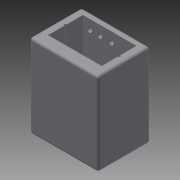
# Autodesk Inventor part: Part1
Saved by Autodesk Inventor 2014 SP1 (Build 180222100, 222)
## iProperties
Created: 2013-12-01
Part Number: Part1
Material: Generic
Document SubType Name: Modeling
Designer: Tim
Density: 1 g/cm^3
Appearance: Default
Author: Tim
Autodesk Inventor part; units mm, degrees
ref_plane "YZ Plane" through (0, 0, 0) normal (1, 0, 0) x (0, 1, 0)
ref_plane "XZ Plane" through (0, 0, 0) normal (0, 1, 0) x (-1, 0, 0)
ref_plane "XY Plane" through (0, 0, 0) normal (0, 0, 1) x (1, 0, 0)
sketch "Sketch1" plane through (0, 0, 0) normal (0, 1, 0) x (-1, 0, 0)
  line L0 (27.4909, -23.2831) -> (-26.5091, -23.2831)
  line L1 (-26.5091, -23.2831) -> (-26.5091, 42.2169)
  line L2 (-26.5091, 42.2169) -> (27.4909, 42.2169)
  line L3 (27.4909, 42.2169) -> (27.4909, -23.2831)
  point P0 (0, 0)
  dimension "d0" = 54
  dimension "d1" = 65.5
  constraints: 8 end point, 2 parallel, 1 horizontal, 1 perpendicular
  measures "d0" distance between parallel lines of L3 L1
  measures "d1" distance between parallel lines of L0 L2
extrude "Extrusion1" add sketch "Sketch1" along normal blind 41
sketch "Sketch2" plane through (-27.4909, 0, 42.2169) normal (0, 0, 1) x (1, 0, 0)
  line L0 (54, 0) -> (0, 0) projected
  line L1 (54, 0) -> (54, 41) projected
  line L2 (0, 41) -> (54, 41) projected
  line L3 (0, 0) -> (0, 41) projected
  line L4 (6, 36) -> (48, 36)
  line L5 (48, 36) -> (48, 5)
  line L6 (48, 5) -> (6, 5)
  line L7 (6, 5) -> (6, 36)
  line L8 (5, 23) -> (49, 23)
  line L9 (49, 23) -> (49, 21.5)
  line L10 (49, 21.5) -> (5, 21.5)
  line L11 (5, 21.5) -> (5, 23)
  point P0 (27.4909, 0)
  dimension "d4" = 42
  dimension "d5" = 31
  dimension "d6" = 5
  dimension "d7" = 6
  dimension "d8" = 6
  dimension "d9" = 1
  dimension "d10" = 1
  dimension "d11" = 13
  dimension "d12" = 1.5
  dimension "d13" = 5
  constraints: 16 end point, 4 parallel, 2 horizontal, 2 perpendicular
  measures "d4" distance between parallel lines of L5 L7
  measures "d5" distance between parallel lines of L6 L4
  measures "d6" distance between parallel lines of L4 L2
  measures "d7" distance between parallel lines of L1 L5
  measures "d8" distance between parallel lines of L3 L7
  measures "d9" distance between parallel lines of L7 L11
  measures "d10" distance between parallel lines of L9 L5
  measures "d11" distance between parallel lines of L4 L8
  measures "d12" distance between parallel lines of L8 L10
  measures "d13" distance between parallel lines of L0 L6
extrude "Extrusion2" cut sketch "Sketch2" against normal blind 60.5 contours L4 L5 L8 L7 | L8 L5 L10 L7 | L7 L10 L11 L8 | L8 L9 L10 L5 | L10 L5 L6 L7
sketch "Sketch3" plane through (0, 41, 0) normal (0, 1, 0) x (1, 0, 0)
  line L0 (26.5091, 23.2831) -> (-27.4909, 23.2831) projected
  line L1 (26.5091, -42.2169) -> (26.5091, 23.2831) projected
  line L2 (-6.9909, -5.7169) -> (18.5091, -5.7169)
  line L3 (18.5091, -5.7169) -> (18.5091, 15.2831)
  line L4 (18.5091, 15.2831) -> (-6.9909, 15.2831)
  line L5 (-6.9909, 15.2831) -> (-6.9909, -5.7169)
  point P0 (0, 0)
  dimension "d16" = 33.5
  dimension "d17" = 29
  dimension "d18" = 8
  dimension "d19" = 8
  constraints: 8 end point, 2 parallel, 1 horizontal, 1 perpendicular
  measures "d16" distance between parallel lines of L1 L5
  measures "d17" distance between parallel lines of L0 L2
  measures "d18" distance between parallel lines of L0 L4
  measures "d19" distance between parallel lines of L1 L3
extrude "Extrusion3" cut sketch "Sketch3" against normal blind 5
sketch "Sketch4" plane through (-21.4909, 5, 42.2169) normal (0, 1, 0) x (1, 0, 0)
  line L0 (0, 0) -> (0, 60.5) projected
  line L1 (0, 8) -> (42, 8)
  line L2 (42, 8) -> (42, 0)
  line L3 (42, 0) -> (0, 0)
  line L4 (0, 0) -> (0, 8)
  point P0 (21.4909, 42.2169)
  dimension "d22" = 8
  constraints: 8 end point, 2 parallel, 1 horizontal, 1 perpendicular, 1 point on line
  measures "d22" distance between parallel lines of L3 L1
extrude "Extrusion4" add sketch "Sketch4" along normal blind 5 separate body
sketch "Sketch5" plane through (0, 41, 0) normal (0, 1, 0) x (1, 0, 0)
  line L0 (26.5091, 23.2831) -> (-27.4909, 23.2831) projected
  line L1 (-27.4909, 23.2831) -> (-27.4909, -42.2169) projected
  circle A0 centre (-16.4909, -34.7169) radius 2
  circle A1 centre (-8.4909, -34.7169) radius 2
  circle A2 centre (0.5091, -34.7169) radius 2
  point P0 (0, 0)
  dimension "d25" = 11
  dimension "d26" = 19
  dimension "d27" = 28
  dimension "d30" = 58
  dimension "d31" = 58
  dimension "d32" = 58
  dimension "d33" = 4
  dimension "d34" = 4
  dimension "d35" = 4
  constraints: 3 centre point
  measures "d25" distance from line of L1 A0.centre
  measures "d26" distance from line of A1.centre L1
  measures "d27" distance from line of A2.centre L1
  measures "d30" distance from line of L0 A0.centre
  measures "d31" distance from line of L0 A1.centre
  measures "d32" distance from line of L0 A2.centre
  measures "d33" diameter of A1
  measures "d34" diameter of A2
  measures "d35" diameter of A0
extrude "Extrusion5" cut sketch "Sketch5" against normal blind 5 bodies 1
fillet "Fillet1" radius 5 1 edges at (-6.9909, 38.5, 5.7169)
fillet "Fillet2" radius 5 1 edges at (18.5091, 38.5, 5.7169)
fillet "Fillet3" radius 2 1 edges at (26.5091, 20.5, -23.2831)
fillet "Fillet4" radius 2 1 edges at (-27.4909, 20.5, -23.2831)
fillet "Fillet5" radius 2 5 edges at (-0.4909, 41, -23.2831) (-26.9051, 41, -22.6973) (-27.4909, 41, 10.4669) (25.9233, 41, -22.6973) (26.5091, 41, 10.4669)
fillet "Fillet6" radius 2 5 edges at (-0.4909, 0, -23.2831) (25.9233, 0, -22.6973) (26.5091, 0, 10.4669) (-26.9051, 0, -22.6973) (-27.4909, 0, 10.4669)
fillet "Fillet7" radius 2 8 edges at (-27.4909, 20.5, 42.2169) (-26.9051, 40.4142, 42.2169) (-0.4909, 41, 42.2169) (25.9233, 40.4142, 42.2169) (26.5091, 20.5, 42.2169) (25.9233, 0.5858, 42.2169) (-0.4909, 0, 42.2169) (-26.9051, 0.5858, 42.2169)
fillet "Fillet8" radius 2 5 edges at (5.7591, 41, 5.7169) (-5.5264, 41, 4.2524) (-6.9909, 41, -7.2831) (17.0446, 41, 4.2524) (18.5091, 41, -7.2831)
fillet "Fillet9" radius 1 3 edges at (-10.4909, 41, 34.7169) (-1.4909, 41, 34.7169) (-18.4909, 41, 34.7169)
fillet "Fillet10" radius 1 3 edges at (-7.9909, 41, -15.2831) (5.7591, 41, -15.2831) (19.5091, 41, -15.2831)
fillet "Fillet11" radius 2 1 edges at (-0.4909, 10, 42.2169)
sketch "Sketch6" plane through (24.5091, 39, -23.2831) normal (0, 0, -1) x (-1, 0, 0)
  line L0 (50, 0) -> (50, -37) projected
  line L1 (0, 0) -> (50, 0) projected
  line L2 (0, -37) -> (0, 0) projected
  line L3 (6, -15) -> (44, -15) construction
  line L4 (44, -15) -> (44, -20) construction
  line L5 (44, -20) -> (6, -20) construction
  line L6 (6, -20) -> (6, -15) construction
  line L7 (7.1714, -18.5227) -> (7.1714, -15.4368)
  line L8 (7.1714, -15.4368) -> (5.9972, -15.4368)
  line L9 (5.9972, -15.4368) -> (5.9972, -15.0227)
  line L10 (5.9972, -15.0227) -> (8.8108, -15.0227)
  line L11 (8.8108, -15.0227) -> (8.8108, -15.4368)
  line L12 (8.8108, -15.4368) -> (7.6365, -15.4368)
  line L13 (7.6365, -15.4368) -> (7.6365, -18.5227)
  line L14 (7.6365, -18.5227) -> (7.1714, -18.5227)
  line L15 (9.5823, -18.5227) -> (9.1398, -18.5227)
  line L16 (9.1398, -18.5227) -> (9.1398, -15.8963)
  line L17 (9.1398, -15.8963) -> (9.5823, -15.8963)
  line L18 (9.5823, -15.8963) -> (9.5823, -18.5227)
  line L19 (9.6135, -15.4595) -> (9.1114, -15.4595)
  line L20 (9.1114, -15.4595) -> (9.1114, -15)
  line L21 (9.1114, -15) -> (9.6135, -15)
  line L22 (9.6135, -15) -> (9.6135, -15.4595)
  spline S0 degree 2 poles (11.2755, -18.5823) (11.0032, -18.5823) (10.5523, -18.4149) (10.3906, -18.2447) knots 0 0 0 1 2 2 2
  spline S1 degree 2 poles (10.3906, -18.2447) (10.2289, -18.0774) (10.0502, -17.5612) (10.0502, -17.2152) knots 0 0 0 1 2 2 2
  spline S2 degree 2 poles (10.0502, -17.2152) (10.0502, -16.8691) (10.2346, -16.3643) (10.3906, -16.1941) knots 0 0 0 1 2 2 2
  spline S3 degree 2 poles (10.3906, -16.1941) (10.5466, -16.0211) (11.0089, -15.8367) (11.2755, -15.8367) knots 0 0 0 1 2 2 2
  spline S4 degree 2 poles (11.2755, -15.8367) (11.4911, -15.8367) (11.8938, -15.9587) (12.0498, -16.0381) knots 0 0 0 1 2 2 2
  line L23 (12.0498, -16.0381) -> (12.0498, -16.5344)
  line L24 (12.0498, -16.5344) -> (12.0243, -16.5344)
  spline S5 degree 2 poles (12.0243, -16.5344) (11.9761, -16.4947) (11.8286, -16.3926) (11.7237, -16.3387) knots 0 0 0 1 2 2 2
  spline S6 degree 2 poles (11.7237, -16.3387) (11.6301, -16.2934) (11.3805, -16.2224) (11.267, -16.2224) knots 0 0 0 1 2 2 2
  spline S7 degree 2 poles (11.267, -16.2224) (10.9238, -16.2224) (10.5069, -16.7415) (10.5069, -17.2152) knots 0 0 0 1 2 2 2
  spline S8 degree 2 poles (10.5069, -17.2152) (10.5069, -17.6775) (10.9096, -18.1965) (11.267, -18.1965) knots 0 0 0 1 2 2 2
  spline S9 degree 2 poles (11.267, -18.1965) (11.4826, -18.1965) (11.874, -18.0178) (12.0243, -17.8788) knots 0 0 0 1 2 2 2
  line L25 (12.0243, -17.8788) -> (12.0498, -17.8788)
  line L26 (12.0498, -17.8788) -> (12.0498, -18.3752)
  spline S10 degree 2 poles (12.0498, -18.3752) (11.9846, -18.4064) (11.7861, -18.4943) (11.7066, -18.5142) knots 0 0 0 1 2 2 2
  spline S11 degree 2 poles (11.7066, -18.5142) (11.5932, -18.5482) (11.4145, -18.5823) (11.2755, -18.5823) knots 0 0 0 1 2 2 2
  line L27 (13.6694, -17.2038) -> (12.3448, -17.2038)
  line L28 (12.3448, -17.2038) -> (12.3448, -16.7784)
  line L29 (12.3448, -16.7784) -> (13.6694, -16.7784)
  line L30 (13.6694, -16.7784) -> (13.6694, -17.2038)
  line L31 (15.0506, -18.5227) -> (15.0506, -15.4368)
  line L32 (15.0506, -15.4368) -> (13.8764, -15.4368)
  line L33 (13.8764, -15.4368) -> (13.8764, -15.0227)
  line L34 (13.8764, -15.0227) -> (16.69, -15.0227)
  line L35 (16.69, -15.0227) -> (16.69, -15.4368)
  line L36 (16.69, -15.4368) -> (15.5158, -15.4368)
  line L37 (15.5158, -15.4368) -> (15.5158, -18.5227)
  line L38 (15.5158, -18.5227) -> (15.0506, -18.5227)
  spline S12 degree 2 poles (18.4741, -18.2447) (18.4202, -18.2844) (18.2387, -18.4263) (18.1536, -18.4688) knots 0 0 0 1 2 2 2
  spline S13 degree 2 poles (18.1536, -18.4688) (18.0373, -18.5312) (17.8189, -18.5964) (17.6203, -18.5964) knots 0 0 0 1 2 2 2
  spline S14 degree 2 poles (17.6203, -18.5964) (17.4587, -18.5964) (17.1665, -18.4745) (17.0559, -18.3639) knots 0 0 0 1 2 2 2
  spline S15 degree 2 poles (17.0559, -18.3639) (16.951, -18.2561) (16.8233, -17.9384) (16.8233, -17.7626) knots 0 0 0 1 2 2 2
  spline S16 degree 2 poles (16.8233, -17.7626) (16.8233, -17.4903) (17.0531, -17.1045) (17.3027, -16.9939) knots 0 0 0 1 2 2 2
  spline S17 degree 2 poles (17.3027, -16.9939) (17.5239, -16.8918) (18.1252, -16.8152) (18.4741, -16.7954) knots 0 0 0 1 2 2 2
  line L39 (18.4741, -16.7954) -> (18.4741, -16.7103)
  spline S18 degree 2 poles (18.4741, -16.7103) (18.4741, -16.5571) (18.3805, -16.3671) (18.2954, -16.3132) knots 0 0 0 1 2 2 2
  spline S19 degree 2 poles (18.2954, -16.3132) (18.2103, -16.2593) (17.9664, -16.2253) (17.8359, -16.2253) knots 0 0 0 1 2 2 2
  spline S20 degree 2 poles (17.8359, -16.2253) (17.6827, -16.2253) (17.2686, -16.316) (17.0616, -16.404) knots 0 0 0 1 2 2 2
  line L40 (17.0616, -16.404) -> (17.0361, -16.404)
  line L41 (17.0361, -16.404) -> (17.0361, -15.953)
  spline S21 degree 2 poles (17.0361, -15.953) (17.158, -15.919) (17.6147, -15.8339) (17.8387, -15.8339) knots 0 0 0 1 2 2 2
  spline S22 degree 2 poles (17.8387, -15.8339) (18.111, -15.8339) (18.4826, -15.919) (18.6301, -16.0296) knots 0 0 0 1 2 2 2
  spline S23 degree 2 poles (18.6301, -16.0296) (18.7747, -16.1374) (18.9165, -16.4806) (18.9165, -16.7273) knots 0 0 0 1 2 2 2
  line L42 (18.9165, -16.7273) -> (18.9165, -18.5227)
  line L43 (18.9165, -18.5227) -> (18.4741, -18.5227)
  line L44 (18.4741, -18.5227) -> (18.4741, -18.2447)
  line L45 (18.4741, -17.876) -> (18.4741, -17.1471)
  spline S24 degree 2 poles (18.4741, -17.1471) (18.3152, -17.1613) (17.8359, -17.2095) (17.6856, -17.2549) knots 0 0 0 1 2 2 2
  spline S25 degree 2 poles (17.6856, -17.2549) (17.5097, -17.3088) (17.28, -17.5328) (17.28, -17.7314) knots 0 0 0 1 2 2 2
  spline S26 degree 2 poles (17.28, -17.7314) (17.28, -17.9583) (17.5353, -18.188) (17.7792, -18.188) knots 0 0 0 1 2 2 2
  spline S27 degree 2 poles (17.7792, -18.188) (17.9862, -18.188) (18.3266, -18.0093) (18.4741, -17.876) knots 0 0 0 1 2 2 2
  spline S28 degree 2 poles (20.5814, -18.5823) (20.3092, -18.5823) (19.8582, -18.4149) (19.6965, -18.2447) knots 0 0 0 1 2 2 2
  spline S29 degree 2 poles (19.6965, -18.2447) (19.5348, -18.0774) (19.3562, -17.5612) (19.3562, -17.2152) knots 0 0 0 1 2 2 2
  spline S30 degree 2 poles (19.3562, -17.2152) (19.3562, -16.8691) (19.5405, -16.3643) (19.6965, -16.1941) knots 0 0 0 1 2 2 2
  spline S31 degree 2 poles (19.6965, -16.1941) (19.8525, -16.0211) (20.3148, -15.8367) (20.5814, -15.8367) knots 0 0 0 1 2 2 2
  spline S32 degree 2 poles (20.5814, -15.8367) (20.797, -15.8367) (21.1998, -15.9587) (21.3558, -16.0381) knots 0 0 0 1 2 2 2
  line L46 (21.3558, -16.0381) -> (21.3558, -16.5344)
  line L47 (21.3558, -16.5344) -> (21.3302, -16.5344)
  spline S33 degree 2 poles (21.3302, -16.5344) (21.282, -16.4947) (21.1345, -16.3926) (21.0296, -16.3387) knots 0 0 0 1 2 2 2
  spline S34 degree 2 poles (21.0296, -16.3387) (20.936, -16.2934) (20.6864, -16.2224) (20.5729, -16.2224) knots 0 0 0 1 2 2 2
  spline S35 degree 2 poles (20.5729, -16.2224) (20.2297, -16.2224) (19.8128, -16.7415) (19.8128, -17.2152) knots 0 0 0 1 2 2 2
  spline S36 degree 2 poles (19.8128, -17.2152) (19.8128, -17.6775) (20.2156, -18.1965) (20.5729, -18.1965) knots 0 0 0 1 2 2 2
  spline S37 degree 2 poles (20.5729, -18.1965) (20.7885, -18.1965) (21.1799, -18.0178) (21.3302, -17.8788) knots 0 0 0 1 2 2 2
  line L48 (21.3302, -17.8788) -> (21.3558, -17.8788)
  line L49 (21.3558, -17.8788) -> (21.3558, -18.3752)
  spline S38 degree 2 poles (21.3558, -18.3752) (21.2905, -18.4064) (21.092, -18.4943) (21.0126, -18.5142) knots 0 0 0 1 2 2 2
  spline S39 degree 2 poles (21.0126, -18.5142) (20.8991, -18.5482) (20.7204, -18.5823) (20.5814, -18.5823) knots 0 0 0 1 2 2 2
  line L50 (22.9753, -17.2038) -> (21.6507, -17.2038)
  line L51 (21.6507, -17.2038) -> (21.6507, -16.7784)
  line L52 (21.6507, -16.7784) -> (22.9753, -16.7784)
  line L53 (22.9753, -16.7784) -> (22.9753, -17.2038)
  line L54 (24.3566, -18.5227) -> (24.3566, -15.4368)
  line L55 (24.3566, -15.4368) -> (23.1823, -15.4368)
  line L56 (23.1823, -15.4368) -> (23.1823, -15.0227)
  line L57 (23.1823, -15.0227) -> (25.9959, -15.0227)
  line L58 (25.9959, -15.0227) -> (25.9959, -15.4368)
  line L59 (25.9959, -15.4368) -> (24.8217, -15.4368)
  line L60 (24.8217, -15.4368) -> (24.8217, -18.5227)
  line L61 (24.8217, -18.5227) -> (24.3566, -18.5227)
  spline S40 degree 2 poles (28.4749, -17.2095) (28.4749, -17.8732) (27.8367, -18.5964) (27.3035, -18.5964) knots 0 0 0 1 2 2 2
  spline S41 degree 2 poles (27.3035, -18.5964) (26.7561, -18.5964) (26.1293, -17.8505) (26.1293, -17.2095) knots 0 0 0 1 2 2 2
  spline S42 degree 2 poles (26.1293, -17.2095) (26.1293, -16.5515) (26.7759, -15.8225) (27.3035, -15.8225) knots 0 0 0 1 2 2 2
  spline S43 degree 2 poles (27.3035, -15.8225) (27.8367, -15.8225) (28.4749, -16.5486) (28.4749, -17.2095) knots 0 0 0 1 2 2 2
  spline S44 degree 2 poles (28.0182, -17.2095) (28.0182, -16.6989) (27.6467, -16.2026) (27.3035, -16.2026) knots 0 0 0 1 2 2 2
  spline S45 degree 2 poles (27.3035, -16.2026) (26.9603, -16.2026) (26.5859, -16.6989) (26.5859, -17.2095) knots 0 0 0 1 2 2 2
  spline S46 degree 2 poles (26.5859, -17.2095) (26.5859, -17.7058) (26.9603, -18.2164) (27.3035, -18.2164) knots 0 0 0 1 2 2 2
  spline S47 degree 2 poles (27.3035, -18.2164) (27.6438, -18.2164) (28.0182, -17.7143) (28.0182, -17.2095) knots 0 0 0 1 2 2 2
  spline S48 degree 2 poles (30.0689, -18.5823) (29.4392, -18.5823) (28.7472, -17.876) (28.7472, -17.2237) knots 0 0 0 1 2 2 2
  spline S49 degree 2 poles (28.7472, -17.2237) (28.7472, -16.5827) (29.4194, -15.8225) (29.9611, -15.8225) knots 0 0 0 1 2 2 2
  spline S50 degree 2 poles (29.9611, -15.8225) (30.205, -15.8225) (30.5823, -15.9643) (30.7212, -16.1147) knots 0 0 0 1 2 2 2
  spline S51 degree 2 poles (30.7212, -16.1147) (30.863, -16.265) (31.0134, -16.6989) (31.0134, -17.0138) knots 0 0 0 1 2 2 2
  line L62 (31.0134, -17.0138) -> (31.0134, -17.2549)
  line L63 (31.0134, -17.2549) -> (29.1953, -17.2549)
  spline S52 degree 2 poles (29.1953, -17.2549) (29.1953, -17.7115) (29.6548, -18.1965) (30.0632, -18.1965) knots 0 0 0 1 2 2 2
  spline S53 degree 2 poles (30.0632, -18.1965) (30.2079, -18.1965) (30.4887, -18.1313) (30.6021, -18.0802) knots 0 0 0 1 2 2 2
  spline S54 degree 2 poles (30.6021, -18.0802) (30.7212, -18.0235) (30.8857, -17.9242) (30.9396, -17.8788) knots 0 0 0 1 2 2 2
  line L64 (30.9396, -17.8788) -> (30.9652, -17.8788)
  line L65 (30.9652, -17.8788) -> (30.9652, -18.361)
  spline S55 degree 2 poles (30.9652, -18.361) (30.8886, -18.3922) (30.656, -18.483) (30.5652, -18.5085) knots 0 0 0 1 2 2 2
  spline S56 degree 2 poles (30.5652, -18.5085) (30.4376, -18.5454) (30.2277, -18.5823) (30.0689, -18.5823) knots 0 0 0 1 2 2 2
  spline S57 degree 2 poles (30.5823, -16.9173) (30.5766, -16.7387) (30.5028, -16.4777) (30.4319, -16.3898) knots 0 0 0 1 2 2 2
  spline S58 degree 2 poles (30.4319, -16.3898) (30.3553, -16.2905) (30.1143, -16.1856) (29.9356, -16.1856) knots 0 0 0 1 2 2 2
  spline S59 degree 2 poles (29.9356, -16.1856) (29.7597, -16.1856) (29.513, -16.2905) (29.4109, -16.3926) knots 0 0 0 1 2 2 2
  spline S60 degree 2 poles (29.4109, -16.3926) (29.3116, -16.4976) (29.2095, -16.75) (29.1953, -16.9173) knots 0 0 0 1 2 2 2
  line L66 (29.1953, -16.9173) -> (30.5823, -16.9173)
  line L67 (35.3189, -18.5227) -> (35.3189, -15.4368)
  line L68 (35.3189, -15.4368) -> (34.1447, -15.4368)
  line L69 (34.1447, -15.4368) -> (34.1447, -15.0227)
  line L70 (34.1447, -15.0227) -> (36.9583, -15.0227)
  line L71 (36.9583, -15.0227) -> (36.9583, -15.4368)
  line L72 (36.9583, -15.4368) -> (35.784, -15.4368)
  line L73 (35.784, -15.4368) -> (35.784, -18.5227)
  line L74 (35.784, -18.5227) -> (35.3189, -18.5227)
  line L75 (37.9652, -18.5227) -> (37.4036, -18.5227)
  line L76 (37.4036, -18.5227) -> (37.4036, -17.8533)
  line L77 (37.4036, -17.8533) -> (37.9652, -17.8533)
  line L78 (37.9652, -17.8533) -> (37.9652, -18.5227)
  line L79 (41.312, -18.5227) -> (40.8468, -18.5227)
  line L80 (40.8468, -18.5227) -> (40.8468, -16.8096)
  line L81 (40.8468, -16.8096) -> (39.2358, -16.8096)
  line L82 (39.2358, -16.8096) -> (39.2358, -18.5227)
  line L83 (39.2358, -18.5227) -> (38.7707, -18.5227)
  line L84 (38.7707, -18.5227) -> (38.7707, -15.0227)
  line L85 (38.7707, -15.0227) -> (39.2358, -15.0227)
  line L86 (39.2358, -15.0227) -> (39.2358, -16.3955)
  line L87 (39.2358, -16.3955) -> (40.8468, -16.3955)
  line L88 (40.8468, -16.3955) -> (40.8468, -15.0227)
  line L89 (40.8468, -15.0227) -> (41.312, -15.0227)
  line L90 (41.312, -15.0227) -> (41.312, -18.5227)
  line L91 (42.6734, -18.5227) -> (42.1118, -18.5227)
  line L92 (42.1118, -18.5227) -> (42.1118, -17.8533)
  line L93 (42.1118, -17.8533) -> (42.6734, -17.8533)
  line L94 (42.6734, -17.8533) -> (42.6734, -18.5227)
  point P0 (24.5091, -39)
  dimension "d49" = 6
  dimension "d50" = 6
  dimension "d51" = 15
  dimension "d52" = 5
  constraints: 2 other
  measures "d49" distance between parallel lines of L2 L6
  measures "d50" distance between parallel lines of L0 L4
  measures "d51" distance between parallel lines of L1 L3
  measures "d52" distance between parallel lines of L3 L5
extrude "Extrusion6" cut sketch "Sketch6" against normal blind 1 bodies 1
equation "\"d31\" = d30"
equation "\"d32\" = d30"
equation "\"d34\" = d33"
equation "\"d35\" = d33"
body "Solid1"
body "Solid2"
